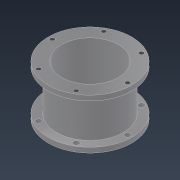
# Autodesk Inventor part: P002-Bati_chambre
Saved by Autodesk Inventor 2021.3 (Build 253353000, 353)
## iProperties
Created: 2022-03-18
Part Number: P002-Bati_chambre
Material: Aluminium
Document SubType Name: Modeling
Designer: Maintenant Prêt
Density: 2.7 g/cm^3
Appearance: Aluminum - Dark
Author: Maintenant Prêt
Autodesk Inventor part; units mm, degrees
ref_plane "YZ Plane" through (0, 0, 0) normal (1, 0, 0) x (0, 1, 0)
ref_plane "XZ Plane" through (0, 0, 0) normal (0, 1, 0) x (-1, 0, 0)
ref_plane "XY Plane" through (0, 0, 0) normal (0, 0, 1) x (1, 0, 0)
sketch "Sketch2" plane through (0, 0, 0) normal (0, 0, 1) x (1, 0, 0)
  line L0 (-28, 0) -> (28, 0) construction
  line L1 (0, -28) -> (0, 28) construction
  circle A0 centre (0, 0) radius 20
  dimension "d3" = 40
  constraints: 1 centre point, 1 coincident
  measures "d3" diameter of A0
extrude "Extrusion1" add sketch "Sketch2" along normal blind 30
sketch "Sketch3" plane through (0, 0, 30) normal (0, 0, 1) x (1, 0, 0)
  point P0 (0, 0)
hole "Hole1" at (0, 0, 30) direction (0, 0, -1) diameter 34 end through all
sketch "Sketch4" plane through (0, 0, 30) normal (0, 0, 1) x (1, 0, 0)
  circle A0 centre (0, 0) radius 20 construction
  circle A1 centre (0, 0) radius 25
  circle A2 centre (0, 0) radius 25 construction
  circle A3 centre (0, 0) radius 20
  circle A4 centre (0, 0) radius 20 construction
  constraints: 2 centre point, 2 coincident, 2 concentric
extrude "Extrusion2" add sketch "Sketch4" against normal blind 3
sketch "Sketch5" plane through (0, 0, 0) normal (0, 0, -1) x (-1, 0, 0)
  circle A0 centre (0, 0) radius 25 construction
  circle A1 centre (0, 0) radius 20 construction
  circle A2 centre (0, 0) radius 25
  circle A3 centre (0, 0) radius 20
  circle A4 centre (0, 0) radius 20 construction
  constraints: 2 centre point, 2 coincident, 2 concentric
extrude "Extrusion3" add sketch "Sketch5" against normal blind 3
sketch "Sketch6" plane through (0, 0, 30) normal (0, 0, 1) x (1, 0, 0)
  circle A0 centre (0, 0) radius 25 construction
  circle A1 centre (0, 0) radius 20 construction
  circle A2 centre (0, 0) radius 22.5 construction
  line L0 (-48.3342, 0) -> (48.3342, 0) construction
  point P0 (-22.5, 0)
  point P1 (-11.25, -19.4856)
  point P2 (11.25, -19.4856)
  point P3 (22.5, 0)
  point P4 (11.25, 19.4856)
  point P5 (-11.25, 19.4856)
  dimension "d19" = 45
  dimension "d17" = 40
  dimension "d18" = 50
  dimension "d22" = 360
  constraints: 2 end point, 1 coincident, 1 horizontal, 1 horizontal alignment, 1 point on line, 11 other
  measures "d17" diameter of A1
  measures "d18" diameter of A0
hole "Hole2" at (-22.5, 0, 30) at (-11.25, -19.4856, 30) at (11.25, -19.4856, 30) at (22.5, 0, 30) at (11.25, 19.4856, 30) at (-11.25, 19.4856, 30) direction (0, 0, -1) diameter 2.459 depth 3 thread size "M3x0.5" class "6H" standard "ISO Metric profile"
sketch "Sketch7" plane through (0, 0, 3) normal (0, 0, 1) x (1, 0, 0)
  circle A0 centre (11.25, -19.4856) radius 1.7 projected
  circle A1 centre (-22.5, 0) radius 1.7 projected
  circle A2 centre (11.25, 19.4856) radius 1.7 projected
  circle A3 centre (-11.25, 19.4856) radius 1.7 projected
  circle A4 centre (-11.25, -19.4856) radius 1.7 projected
  circle A5 centre (22.5, 0) radius 1.7 projected
  circle A6 centre (0, 0) radius 20 projected
  circle A7 centre (0, 0) radius 25 projected
hole "Hole3" at (11.25, -19.4856, 3) at (22.5, 0, 3) at (11.25, 19.4856, 3) at (-11.25, 19.4856, 3) at (-22.5, 0, 3) at (-11.25, -19.4856, 3) direction (0, 0, -1) diameter 3.4 depth 3 clearance for "Flat Head Machine Screw" size "M3" standard "Ansi Metric M Profile"
equation "\"d19\" = 0.5 * d18 + 0.5 * d17"
body "Solid1"
